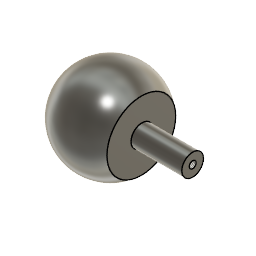
BRASPOURGLISSIERE1 (Autodesk Fusion 360 design; units mm, degrees)
Autodesk Fusion 360 part; units mm, degrees
sphere "SpherePrimitive1" add diameter 34 placed x (0, 1, 0) y (0, 0, 1) z (1, 0, 0) at (0, 0, 0)
cylinder "CylindrePrimitive1" add diameter 8 height 30 placed x (0, 0, -1) y (0, 1, 0) z (1, 0, 0) at (0, 0.2086, 0)
cylinder "CylindrePrimitive2" add diameter 3 height 4 placed x (0, 0, -1) y (0, 1, 0) z (1, 0, 0) at (30, 0, 0)
thread "Filetage1" "ISO Metric profile 3.0 M3x0.5 M3x0.5 6g" major diameter 2.927 minor diameter 2.3555 pitch 0.5 angle 60 resizes the face on face at (32.6667, -0.1494, -1.4925)
delete_face "DeleteFace1" 1 faces at (32.6667, -0.1457, -1.4562)
hole "Perçage1" at (30, 0.2086, 0) direction (-1, 0, 0) diameter 2.529 depth 4 tip angle 118
thread "Filetage2" "ISO Metric profile 3.0 M3x0.5 M3x0.5 6H" major diameter 3.086 minor diameter 2.529 pitch 0.5 angle 60 resizes the face on face at (27.3333, 0.3345, -1.2582)
delete_face "DeleteFace2" 1 faces at (27.3333, 0.3345, -1.2582)
hole "Perçage2" at (30, 0.2086, 0) direction (-1, 0, 0) diameter 2.529 depth 6 tip angle 118
thread "Filetage3" "ISO Metric profile 3.0 M3x0.5 M3x0.5 6H" thread offset 0 thread depth 7.4
sketch "Esquisse4" plane through (30, 0, 0) normal (1, 0, 0) x (0, 1, 0)
  circle A0 centre (0.2086, 0) radius 1.2645
  circle A1 centre (0.2086, 0) radius 4
  circle A2 centre (0.2086, 0) radius 19.105
  constraint concentric A0 A2
extrude "Extrusion1" cut sketch "Esquisse4" against normal blind 18.6 contours A2
